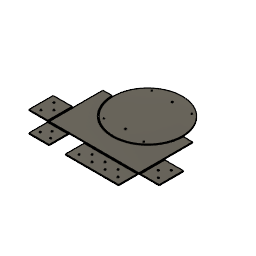
reflow-plate (Autodesk Fusion 360 design; units mm, degrees)
part number: 2025-12-24-11-57-15-769
Autodesk Fusion 360 part; units mm, degrees
note: some values were not read from the file. Set by a fixed rule: which sketch regions a step uses.
sketch "Sketch1" plane through (0, 0, 0) normal (0, 0, 1) x (1, 0, 0)
  circle A0 centre (0, 0) radius 85
  line L0 (110.5, -132.5) -> (-110.5, -132.5)
  line L1 (-110.5, -132.5) -> (-110.5, 0)
  line L2 (110.5, 0) -> (110.5, -132.5)
  line L3 (110.5, -132.5) -> (-110.5, 132.5) construction
  line L4 (-110.5, -132.5) -> (110.5, 132.5) construction
  line L5 (110.5, -132.5) -> (160.5, -132.5)
  line L6 (160.5, -132.5) -> (160.5, -72.5)
  line L7 (160.5, -72.5) -> (110.5, -72.5)
  line L8 (-110.5, -132.5) -> (-160.5, -132.5)
  line L9 (-160.5, -132.5) -> (-160.5, -72.5)
  line L10 (-160.5, -72.5) -> (-110.5, -72.5)
  line L11 (110.5, -132.5) -> (110.5, -182.5)
  line L12 (110.5, -182.5) -> (60.5, -182.5)
  line L13 (60.5, -182.5) -> (60.5, -132.5)
  line L14 (60.5, -132.5) -> (20.5, -132.5)
  line L15 (20.5, -132.5) -> (20.5, -182.5)
  line L16 (-110.5, -132.5) -> (-110.5, -182.5)
  line L17 (-110.5, -182.5) -> (20.5, -182.5)
  line L18 (110.5, 0) -> (87.5, 0)
  line L19 (-87.5, 0) -> (-110.5, 0)
  arc A1 (-87.5, 0) -> (87.5, 0) centre (0, 0) ccw
  circle A2 centre (49.3161, 59.1347) radius 1.6
  line L20 (48.3908, 70.3233) -> (63.1359, 58.0265)
  circle A3 centre (-49.3161, 59.1347) radius 1.6
  line L21 (-46.7429, 71.6976) -> (-62.5753, 58.494)
  line L22 (64.1541, -57.1773) -> (44.5743, -73.5061)
  circle A4 centre (49.3161, -59.1347) radius 1.6
  circle A5 centre (-49.639, -59.5218) radius 1.6
  line L23 (-65.6875, -58.5548) -> (-44.1612, -72.6889)
  line L24 (110.5, -72.5) -> (113.7, -72.5)
  line L25 (113.7, -72.5) -> (113.7, -132.5)
  line L26 (113.7, -132.5) -> (110.5, -132.5)
  line L27 (110.5, -132.5) -> (110.5, -72.5)
  line L28 (110.5, -132.5) -> (-110.5, -132.5)
  line L29 (-110.5, -132.5) -> (-110.5, -135.7)
  line L30 (110.5, -135.7) -> (110.5, -132.5)
  line L31 (-110.5, -72.5) -> (-113.7, -72.5)
  line L32 (-113.7, -72.5) -> (-113.7, -132.5)
  line L33 (-113.7, -132.5) -> (-110.5, -132.5)
  line L34 (-110.5, -132.5) -> (-110.5, -72.5)
  line L35 (0, 60) -> (0, -55)
  circle A6 centre (0, 60) radius 2
  circle A7 centre (0, -55) radius 2
  line L36 (144.5, -72.5) -> (144.5, -132.5)
  line L37 (128.5, -72.5) -> (128.5, -132.5)
  line L38 (-144.5, -72.5) -> (-144.5, -132.5)
  line L39 (110.5, -150.5) -> (60.5, -150.5)
  line L40 (20.5, -150.5) -> (-110.5, -150.5)
  line L41 (110.5, -166.5) -> (60.5, -166.5)
  line L42 (20.5, -166.5) -> (-110.5, -166.5)
  line L43 (-128.5, -72.5) -> (-128.5, -132.5)
  circle A8 centre (144.5, -86.5) radius 2
  circle A9 centre (128.5, -102.5) radius 2
  circle A10 centre (144.5, -118.5) radius 2
  circle A11 centre (98.5, -166.5) radius 2
  circle A12 centre (85.5, -150.5) radius 2
  circle A13 centre (72.5, -166.5) radius 2
  circle A14 centre (3, -166.5) radius 2
  circle A15 centre (-29, -166.5) radius 2
  circle A16 centre (-13, -150.5) radius 2
  circle A17 centre (-45, -150.5) radius 2
  circle A18 centre (-77, -150.5) radius 2
  circle A19 centre (-61, -166.5) radius 2
  circle A20 centre (-93, -166.5) radius 2
  circle A21 centre (-144.5, -86.5) radius 2
  circle A22 centre (-144.5, -118.5) radius 2
  circle A23 centre (-128.5, -102.5) radius 2
  line L44 (-110.5, -135.7) -> (20.5, -135.7)
  line L45 (60.5, -135.7) -> (110.5, -135.7)
  dimension "d1" = 170
  dimension "d2" = 175
  dimension "d3" = 132.5
  dimension "d4" = 221
  dimension "d5" = 50
  dimension "d6" = 60
  dimension "d7" = 50
  dimension "d8" = 60
  dimension "d9" = 50
  dimension "d10" = 50
  dimension "d11" = 40
  dimension "d12" = 50
  dimension "d13" = 50
  dimension "d14" = 3.2
  dimension "d15" = 8
  dimension "d16" = 8
  dimension "d17" = 3.2
  dimension "d18" = 8
  dimension "d19" = 3.2
  dimension "d20" = 8
  dimension "d23" = 3.2
  dimension "d24" = 3.2
  dimension "d25" = 3.2
  dimension "d28" = 115
  dimension "d29" = 60
  dimension "d30" = 4
  dimension "d31" = 4
  dimension "d36" = 16
  dimension "d37" = 16
  dimension "d38" = 16
  dimension "d39" = 16
  dimension "d40" = 16
  dimension "d41" = 16
  dimension "d42" = 4
  dimension "d43" = 4
  dimension "d44" = 4
  dimension "d45" = 110.5
  dimension "d46" = 14
  dimension "d47" = 14
  dimension "d48" = 30
  dimension "d49" = 4
  dimension "d50" = 4
  dimension "d51" = 4
  dimension "d52" = 12
  dimension "d53" = 12
  dimension "d54" = 4
  dimension "d55" = 4
  dimension "d59" = 4
  dimension "d60" = 4
  dimension "d61" = 4
  dimension "d63" = 17.5
  dimension "d64" = 32
  dimension "d67" = 4
  dimension "d68" = 32
  dimension "d69" = 4
  dimension "d70" = 32
  dimension "d71" = 32
  dimension "d72" = 32
  dimension "d73" = 33.5
  dimension "d74" = 4
  dimension "d75" = 14
  dimension "d76" = 4
  dimension "d77" = 32
  dimension "d78" = 4
  dimension "d79" = 30
  constraint coincident A0.centre A1.centre
  constraint horizontal L0
  constraint perpendicular L0 L1
  constraint parallel L1 L2
  constraint coincident L3 A0.centre
  constraint coincident L4 A0.centre
  constraint perpendicular L2 L5
  constraint perpendicular L5 L6
  constraint coincident L2 L7.end
  constraint perpendicular L2 L7
  constraint perpendicular L1 L8
  constraint perpendicular L8 L9
  constraint coincident L1 L10.end
  constraint perpendicular L1 L10
  constraint perpendicular L0 L11
  constraint perpendicular L11 L12
  constraint coincident L0 L13.end
  constraint perpendicular L0 L13
  constraint perpendicular L13 L14
  constraint perpendicular L0 L15
  constraint perpendicular L0 L16
  constraint perpendicular L2 L18
  constraint perpendicular L1 L19
  constraint coincident L4 A2.centre
  constraint perpendicular L4 L20
  constraint tangent A0 L20
  constraint coincident L3 A3.centre
  constraint equal A2 A3
  constraint perpendicular L3 L21
  constraint tangent A0 L21
  constraint perpendicular L3 L22
  constraint tangent A0 L22
  constraint coincident L3 A4.centre
  constraint coincident L4 A5.centre
  constraint tangent A0 L23
  constraint horizontal L24
  constraint vertical L25
  constraint horizontal L26
  constraint vertical L27
  constraint horizontal L28
  constraint vertical L29
  constraint horizontal L44
  constraint vertical L30
  constraint horizontal L31
  constraint vertical L32
  constraint horizontal L33
  constraint vertical L34
  constraint vertical L35
  constraint coincident L35.start A6.centre
  constraint coincident L35.end A7.centre
  constraint coincident L7 L36.start
  constraint coincident L5 L36.end
  constraint perpendicular L5 L36
  constraint coincident L7 L37.start
  constraint coincident L5 L37.end
  constraint perpendicular L5 L37
  constraint coincident L11 L41.start
  constraint coincident L16 L42.end
  constraint perpendicular L16 L41
  constraint coincident L11 L39.start
  constraint coincident L16 L40.end
  constraint perpendicular L16 L39
  constraint coincident L10 L38.start
  constraint coincident L8 L38.end
  constraint perpendicular L8 L38
  constraint coincident L13 L39.end
  constraint coincident L15 L40.start
  constraint collinear L39 L40
  constraint coincident L13 L41.end
  constraint coincident L15 L42.start
  constraint collinear L41 L42
  constraint coincident L10 L43.start
  constraint coincident L8 L43.end
  constraint perpendicular L8 L43
  constraint coincident L36 A8.centre
  constraint coincident L37 A9.centre
  constraint coincident L36 A10.centre
  constraint coincident L41 A11.centre
  constraint midpoint L39 A12.centre
  constraint coincident L41 A13.centre
  constraint coincident L42 A14.centre
  constraint coincident L42 A15.centre
  constraint coincident L40 A16.centre
  constraint coincident L40 A17.centre
  constraint coincident L40 A18.centre
  constraint coincident L42 A19.centre
  constraint coincident L42 A20.centre
  constraint coincident L38 A21.centre
  constraint coincident L38 A22.centre
  constraint coincident L43 A23.centre
  constraint coincident L15 L44.end
  constraint coincident L13 L45.start
  constraint collinear L44 L45
  measures "d1" diameter of A0
  measures "d2" diameter of A1
  measures "d3" distance of A0.centre L0
  measures "d4" distance of L1 L2
  measures "d5" distance of L0.start L5.end
  measures "d6" distance of L5.end L6.end
  measures "d7" distance of L0.end L8.end
  measures "d8" distance of L8.end L9.end
  measures "d9" distance of L0.start L11.end
  measures "d10" distance of L11.end L12.end
  measures "d11" distance of L13.end L14.end
  measures "d12" distance of L14.end L15.end
  measures "d13" distance of L0.end L16.end
  measures "d14" diameter of A2
  measures "d15" distance of A2.centre L20
  measures "d16" distance of A3.centre L21
  measures "d17" diameter of A4
  measures "d18" distance of L22 A4.centre
  measures "d19" diameter of A5
  measures "d20" distance of A5.centre L23
  measures "d23" distance of L7.end L24.end
  measures "d24" distance of L0.start L30.start
  measures "d25" distance of L10.end L31.end
  measures "d28" distance of L35.start L35.end
  measures "d29" distance of A0.centre L35.start
  measures "d30" diameter of A6
  measures "d31" diameter of A7
  measures "d36" distance of L6 L36
  measures "d37" distance of L36 L37
  measures "d38" distance of L12 L41
  measures "d39" distance of L39 L41
  measures "d40" distance of L9 L38
  measures "d41" distance of L38 L43
  measures "d42" diameter of A8
  measures "d43" diameter of A9
  measures "d44" diameter of A10
  measures "d45" distance of A0.centre L2.start
  measures "d46" distance of L36.start A8.centre
  measures "d47" distance of L36.end A10.centre
  measures "d48" distance of L37.start A9.centre
  measures "d49" diameter of A11
  measures "d50" diameter of A12
  measures "d51" diameter of A13
  measures "d52" distance of L11 A11.centre
  measures "d53" distance of L13 A13.centre
  measures "d54" diameter of A14
  measures "d55" diameter of A15
  measures "d59" diameter of A16
  measures "d60" diameter of A17
  measures "d61" diameter of A18
  measures "d63" distance of L42.start A14.centre
  measures "d64" distance of A14.centre A15.centre
  measures "d67" diameter of A19
  measures "d68" distance of A15.centre A19.centre
  measures "d69" diameter of A20
  measures "d70" distance of A19.centre A20.centre
  measures "d71" distance of A16.centre A17.centre
  measures "d72" distance of A17.centre A18.centre
  measures "d73" distance of L40.start A16.centre
  measures "d74" diameter of A21
  measures "d75" distance of L38.start A21.centre
  measures "d76" diameter of A22
  measures "d77" distance of A21.centre A22.centre
  measures "d78" diameter of A23
  measures "d79" distance of L43.start A23.centre
extrude "Extrude1" add sketch "Sketch1" along normal blind 2 contours A0 | L0 L11 L13 L28 L30 L45 | L0 L1 L2 L14 L18 L19 A1 L27 L28 L34 | L2 L5 L7 L24 L25 L26 L27 | L5 L7 L25 L37 A9 | L11 L13 L39 A12 L45 | L0 L15 L16 L28 L29 L44 | L5 L7 L36 L37 A8 A9 A10 | L11 L13 L39 L41 A11 A12 A13 | L1 L8 L10 L31 L32 L33 L34 | L15 L16 L40 A16 A17 A18 L44 | L5 L6 L7 L36 A8 A10 | L37 A9 | L37 A9 | L11 L12 L13 L41 A11 A13 | L39 A12 | L39 A12 | L8 L10 L32 L43 A23 | L15 L16 L40 L42 A14 A15 A16 A17 A18 A19 A20 | L36 A10 | L36 A10 | L41 A11 | L41 A11 | L8 L10 L38 L43 A21 A22 A23 | L15 L16 L17 L42 A14 A15 A19 A20 | L40 A16 | L40 A16 | L41 A13 | L41 A13 | L36 A8 | L36 A8 | L8 L9 L10 L38 A21 A22 | L43 A23 | L43 A23 | L40 A18 | L40 A18 | L42 A14 | L42 A14 | L38 A22 | L38 A22 | L42 A20 | L42 A20 | L40 A17 | L40 A17 | L38 A21 | L38 A21 | L42 A15 | L42 A15 | L42 A19 | L42 A19 | A6 | A7 makes body 1 at (-36.4902, -116.7687, 0) makes body 2 at (-16.2722, -19.4779, 0)
extrude "Extrude2" cut sketch "Sketch1" along normal blind 0.5 contours L0 L11 L13 L28 L30 L45 | L2 L5 L7 L24 L25 L26 L27 | L0 L15 L16 L28 L29 L44 | L1 L8 L10 L31 L32 L33 L34 bodies 1
extrude "Extrude3" cut sketch "Sketch1" along normal blind 2 contours A6 | A7 bodies 2
extrude "Extrude4" cut sketch "Sketch1" along normal blind 2 contours L37 A9 | L37 A9 | L39 A12 | L39 A12 | L36 A10 | L36 A10 | L41 A11 | L41 A11 | L40 A16 | L40 A16 | L41 A13 | L41 A13 | L36 A8 | L36 A8 | L43 A23 | L43 A23 | L40 A18 | L40 A18 | L42 A14 | L42 A14 | L38 A22 | L38 A22 | L42 A20 | L42 A20 | L40 A17 | L40 A17 | L38 A21 | L38 A21 | L42 A15 | L42 A15 | L42 A19 | L42 A19 bodies 1
move_body "Move1" bodies 2 1 to x (-1, 0, 0) y (0, 1, 0) z (0, 0, -1) at (0, 0, 0)
move_body "Move2" bodies 2 1 to x (1, 0, 0) y (0, 1, 0) z (0, 0, 1) at (0, 0, 2)
equation "d3 = ( 185 mm / 2 ) + 40 mm"
